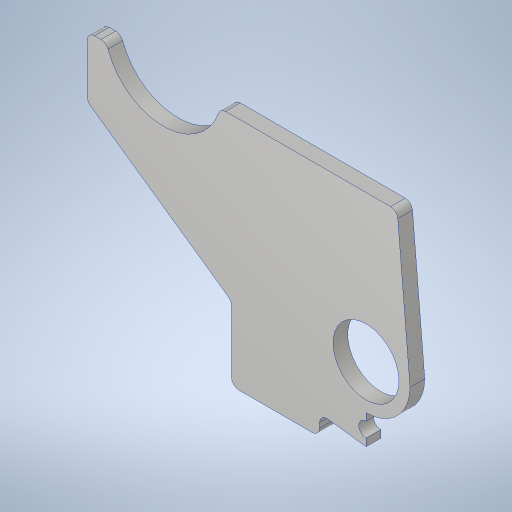
# Autodesk Inventor part: CL1-002
Saved by Autodesk Inventor 2023.4 (Build 274418000, 418)
## iProperties
Created: 2025-01-17
Part Number: CL1-002
Material: Aluminum 6061
Document SubType Name: Modeling
Designer: mavericks
Density: 2.7 g/cm^3
Appearance: Aluminum - Flat
Author: mavericks
Autodesk Inventor part; units mm, degrees
ref_plane "YZ Plane" through (0, 0, 0) normal (1, 0, 0) x (0, 1, 0)
ref_plane "XZ Plane" through (0, 0, 0) normal (0, 1, 0) x (-1, 0, 0)
ref_plane "XY Plane" through (0, 0, 0) normal (0, 0, 1) x (1, 0, 0)
sketch "Sketch1" plane through (0, 0, 0) normal (0, 0, 1) x (1, 0, 0)
  line L0 (-69.85, -50.8) -> (69.85, -50.8) construction
  line L1 (69.85, -50.8) -> (69.85, 50.8) construction
  line L2 (69.85, 50.8) -> (-69.85, 50.8) construction
  line L3 (-69.85, 50.8) -> (-69.85, -50.8) construction
  line L4 (-69.85, -50.8) -> (69.85, 50.8) construction
  line L5 (69.85, -50.8) -> (-69.85, 50.8) construction
  circle A0 centre (-36.9364, 57.15) radius 25.4 construction
  circle A1 centre (50.8, -12.7) radius 14.2875 construction
  circle A2 centre (50.8, -12.7) radius 19.05 construction
  line L6 (-69.85, 24.6565) -> (-7.4306, -19.05) construction
  line L7 (-7.4306, -19.05) -> (-7.4306, -50.8) construction
  line L8 (30.6694, -50.8) -> (30.6694, -41.91) construction
  line L9 (30.6694, -41.91) -> (50.8, -38.1) construction
  line L10 (50.8, -38.1) -> (50.8, -31.75) construction
  line L11 (69.85, -12.7) -> (64.2945, 50.8) construction
  line L12 (-7.4306, -50.8) -> (30.6694, -50.8)
  line L13 (30.6694, -50.8) -> (30.6694, -41.91)
  line L14 (50.8, -38.1) -> (50.8, -31.75)
  line L15 (69.85, -12.7) -> (64.2945, 50.8)
  line L16 (64.2945, 50.8) -> (-12.343, 50.8)
  line L17 (-69.85, 50.8) -> (-61.5299, 50.8)
  line L18 (-69.85, 50.8) -> (-69.85, 24.6565)
  line L19 (-69.85, 24.6565) -> (-7.4306, -19.05)
  line L20 (-7.4306, -19.05) -> (-7.4306, -50.8)
  circle A3 centre (50.8, -12.7) radius 14.2875
  arc A4 (-61.5299, 50.8) -> (-12.343, 50.8) centre (-36.9364, 57.15) ccw
  circle A5 centre (50.8, -38.1) radius 3.175
  arc A6 (50.8, -31.75) -> (69.85, -12.7) centre (50.8, -12.7) ccw
  line L21 (50.8, -38.1) -> (50.8, -44.5024)
  line L22 (50.8, -44.5024) -> (30.6694, -41.91)
  point P0 (0, 0)
  point P1 (50.8, -34.925)
  point P2 (50.8, -41.275)
  dimension "d0" = 101.6
  dimension "d1" = 139.7
  dimension "d3" = 50.8
  dimension "d4" = 6.35
  dimension "d5" = 36.9364
  dimension "d6" = 19.05
  dimension "d7" = 38.1
  dimension "d8" = 38.1
  dimension "d9" = 28.575
  dimension "d10" = 125
  dimension "d11" = 31.75
  dimension "d12" = 76.2
  dimension "d15" = 8.89
  dimension "d17" = 38.1
  dimension "d18" = 95
  dimension "d25" = 6.35
  dimension "d26" = 25.4
  dimension "d28" = 4.7625
  dimension "d31" = 6.35
  constraints: 46 end point, 8 point on circle, 8 point on line, 7 centre point, 6 collinear, 4 coincident, 4 perpendicular, 3 parallel, 2 midpoint, 1 concentric, 1 horizontal, 1 vertical, 1 vertical alignment
  measures "d0" distance of L0.end L1.end
  measures "d1" distance of L1.end L2.end
  measures "d3" diameter of A0
  measures "d4" vertical distance of L2.end A0.centre
  measures "d5" horizontal distance of point (0, 0) A0.centre
  measures "d6" distance from line of L1 A1.centre
  measures "d7" distance from line of L0 A1.centre
  measures "d8" diameter of A2
  measures "d9" diameter of A1
  measures "d10" angle of L7 L6
  measures "d11" distance of L6.end L7.end
  measures "d12" distance of L6.start L6.end
  measures "d15" distance of L8.start L8.end
  measures "d17" distance between parallel lines of L13 L7
  measures "d18" angle of L16 L15
  measures "d25" diameter of A5
  measures "d26" distance of L21.start A1.centre
  measures "d28" radial gap between concentric circles of A2 A3
  measures "d31" distance from line of L21.start L22
extrude "Extrusion1" add sketch "Sketch1" along normal blind 6.35 contours L20 L19 L18 L17 A4 L16 L15 A6 L14 A5 L21 L22 L13 L12
fillet "Fillet1" radius 3.175 9 edges at (-7.4306, -50.8, 3.175) (30.6694, -50.8, 3.175) (30.6694, -41.91, 3.175) (64.2945, 50.8, 3.175) (-12.343, 50.8, 3.175) (-61.5299, 50.8, 3.175) (-69.85, 50.8, 3.175) (-69.85, 24.6565, 3.175) (-7.4306, -19.05, 3.175)
body "Solid1"
